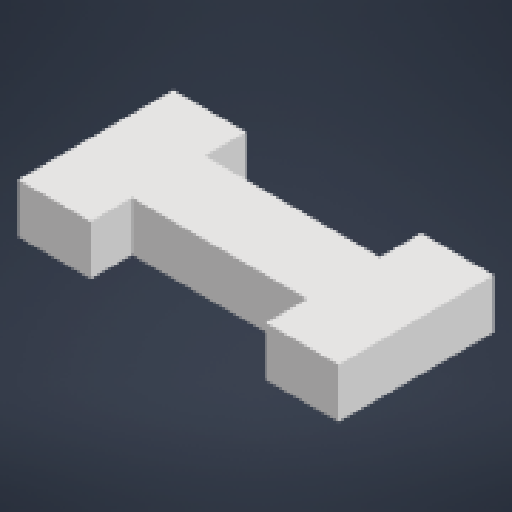
# Autodesk Inventor part: 3mmPin
Saved by Autodesk Inventor 2026 (Build 300175050, 175E)
## iProperties
Created: 2026-04-30
Part Number: 3mmPin
Material: Generic
Document SubType Name: Modeling
Designer: sniel
Density: 1 g/cm^3
Appearance: Default
Author: sniel
Autodesk Inventor part; units mm, degrees
ref_plane "YZ Plane" through (0, 0, 0) normal (1, 0, 0) x (0, 1, 0)
ref_plane "XZ Plane" through (0, 0, 0) normal (0, 1, 0) x (-1, 0, 0)
ref_plane "XY Plane" through (0, 0, 0) normal (0, 0, 1) x (1, 0, 0)
sketch "Sketch1" plane through (0, 0, 0) normal (0, 1, 0) x (-1, 0, 0)
  line L0 (15, -7.2) -> (15, 2.5)
  line L1 (15, 2.5) -> (10.3, 2.5)
  line L2 (10.3, 0) -> (10.3, 2.5)
  line L3 (10.3, 0) -> (0, 0)
  line L4 (0, 0) -> (0, 2.5)
  line L5 (0, 2.5) -> (-4.7, 2.5)
  line L6 (-4.7, 2.5) -> (-4.7, -7.2)
  line L7 (-4.7, -7.2) -> (0, -7.2)
  line L8 (0, -7.2) -> (0, -4.7)
  line L9 (0, -4.7) -> (10.3, -4.7)
  line L10 (10.3, -7.2) -> (10.3, -4.7)
  line L11 (15, -7.2) -> (10.3, -7.2)
  line L12 (15, 2.5) -> (14.85, 2.5)
  line L13 (14.85, 2.5) -> (14.85, 2.35)
  line L14 (14.85, 2.35) -> (15, 2.35)
  line L15 (15, 2.35) -> (15, 2.5)
  line L16 (10.3, -7.2) -> (10.45, -7.2)
  line L17 (10.45, -7.2) -> (10.45, -7.05)
  line L18 (10.45, -7.05) -> (10.3, -7.05)
  line L19 (10.3, -7.05) -> (10.3, -7.2)
  line L20 (0, 2.5) -> (-0.15, 2.5)
  line L21 (-0.15, 2.5) -> (-0.15, 2.35)
  line L22 (-0.15, 2.35) -> (0, 2.35)
  line L23 (0, 2.35) -> (0, 2.5)
  line L24 (-4.7, -7.2) -> (-4.55, -7.2)
  line L25 (-4.55, -7.2) -> (-4.55, -7.05)
  line L26 (-4.55, -7.05) -> (-4.7, -7.05)
  line L27 (-4.7, -7.05) -> (-4.7, -7.2)
  line L28 (-0.15, 2.35) -> (-4.55, 2.35)
  line L29 (-4.55, 2.35) -> (-4.55, -7.05)
  line L30 (-4.55, -7.05) -> (-0.15, -7.05)
  line L31 (-0.15, -7.05) -> (-0.15, 2.35)
  line L32 (14.85, 2.35) -> (10.45, 2.35)
  line L33 (10.45, 2.35) -> (10.45, -7.05)
  line L34 (10.45, -7.05) -> (14.85, -7.05)
  line L35 (14.85, -7.05) -> (14.85, 2.35)
  line L36 (10.45, 0) -> (10.3, 0)
  line L37 (10.3, 0) -> (10.3, -0.15)
  line L38 (10.3, -0.15) -> (10.45, -0.15)
  line L39 (10.45, -0.15) -> (10.45, 0)
  line L40 (0, -4.7) -> (-0.15, -4.7)
  line L41 (-0.15, -4.7) -> (-0.15, -4.55)
  line L42 (-0.15, -4.55) -> (0, -4.55)
  line L43 (0, -4.55) -> (0, -4.7)
  line L44 (-0.15, -4.55) -> (10.45, -4.55)
  line L45 (10.45, -4.55) -> (10.45, -0.15)
  line L46 (10.45, -0.15) -> (-0.15, -0.15)
  line L47 (-0.15, -0.15) -> (-0.15, -4.55)
  point P0 (0, 0)
  point P1 (-0.15, -0.15)
  dimension "d2" = 0.15
  dimension "d3" = 0.15
  dimension "d4" = 0.15
  dimension "d5" = 0.15
  dimension "d6" = 0.15
  dimension "d7" = 0.15
  dimension "d8" = 0.15
  dimension "d9" = 0.15
  dimension "d10" = 0.15
  dimension "d11" = 0.15
  dimension "d12" = 0.15
  dimension "d13" = 0.15
  constraints: 96 end point, 18 parallel, 9 horizontal, 9 perpendicular, 1 point on line
  measures "d2" distance of L14.end L13.end
  measures "d3" distance of L13.end L12.end
  measures "d4" distance of L18.end L17.end
  measures "d5" distance of L17.end L16.end
  measures "d6" distance of L22.end L21.end
  measures "d7" distance of L21.end L20.end
  measures "d8" distance of L26.end L25.end
  measures "d9" distance of L25.end L24.end
  measures "d10" distance of L38.end L37.end
  measures "d11" distance of L37.end L36.end
  measures "d12" distance of L41.end L42.end
  measures "d13" distance of L40.end L41.end
extrude "Extrusion1" add sketch "Sketch1" along normal blind 3 contours L35 L34 L33 L32 | L44 L42 L31 L46 L38 L33 | L31 L30 L29 L28
body "Solid1"
